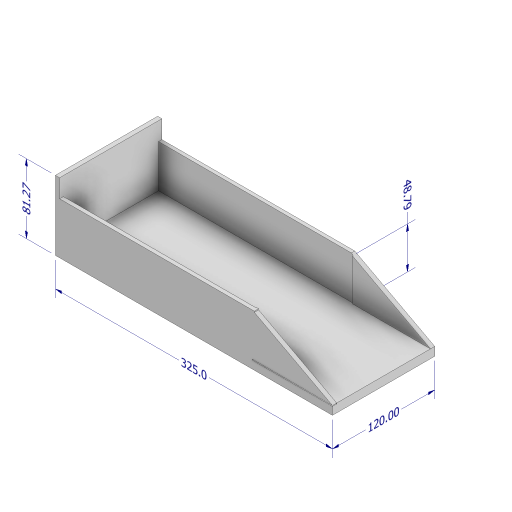
# Autodesk Inventor part: Storagecontainer
Saved by Autodesk Inventor 2024 (Build 280153000, 153)
## iProperties
Created: 2023-05-30
Part Number: Storagecontainer
Material: Generic
Document SubType Name: Modeling
Designer: Lenovo
Density: 1 g/cm^3
Appearance: Default
Author: Lenovo
Autodesk Inventor part; units mm, degrees
ref_plane "YZ Plane" through (0, 0, 0) normal (1, 0, 0) x (0, 1, 0)
ref_plane "XZ Plane" through (0, 0, 0) normal (0, 1, 0) x (-1, 0, 0)
ref_plane "XY Plane" through (0, 0, 0) normal (0, 0, 1) x (1, 0, 0)
sketch "Sketch1" plane through (0, 0, 0) normal (0, 1, 0) x (-1, 0, 0)
  line L0 (-160, 60) -> (160, 60)
  line L1 (160, 60) -> (160, -60)
  line L2 (160, -60) -> (-160, -60)
  line L3 (-160, -60) -> (-160, 60)
  line L4 (-160, 60) -> (160, -60) construction
  line L5 (160, 60) -> (-160, -60) construction
  line L6 (-27.6343, -87.1189) -> (-42.3128, -87.1189)
  line L7 (-42.3128, -87.1189) -> (-42.3128, -133.601)
  line L8 (-42.3128, -133.601) -> (-27.6343, -133.601)
  line L9 (-27.6343, -133.601) -> (-27.6343, -87.1189)
  line L10 (-27.6343, -87.1189) -> (-42.3128, -133.601) construction
  line L11 (-42.3128, -87.1189) -> (-27.6343, -133.601) construction
  point P0 (0, 0)
  point P1 (-34.9736, -110.3599)
  dimension "d0" = 320
  dimension "d1" = 120
  constraints: 24 end point, 4 midpoint, 4 parallel, 2 horizontal, 2 perpendicular
  measures "d0" distance of L1.end L2.end
  measures "d1" distance of L0.end L1.end
extrude "Extrusion1" add sketch "Sketch1" along normal blind 10 contours L0 L1 L2 L3
sketch "Sketch2" plane through (0, 10, 0) normal (0, 1, 0) x (1, 0, 0)
  line L0 (-160, -60) -> (160, -60) projected
  line L1 (-160, -60) -> (66.1592, -60)
  line L2 (66.1592, -60) -> (66.1592, -55.6043)
  line L3 (66.1592, -55.6043) -> (-160, -55.6043)
  line L4 (-160, -55.6043) -> (-160, -60)
  point P0 (0, 0)
  constraints: 8 end point, 2 parallel, 1 horizontal, 1 perpendicular
extrude "Extrusion2" add sketch "Sketch2" along normal blind 50
sketch "Sketch3" plane through (0, 10, 0) normal (0, 1, 0) x (1, 0, 0)
  line L0 (-160, 60) -> (-160, -60) projected
  line L1 (-160, 60) -> (68.4346, 60)
  line L2 (68.4346, 60) -> (68.4346, 56.0614)
  line L3 (68.4346, 56.0614) -> (-160, 56.0614)
  line L4 (-160, 56.0614) -> (-160, 60)
  point P0 (0, 0)
  constraints: 8 end point, 2 parallel, 1 horizontal, 1 perpendicular
extrude "Extrusion3" add sketch "Sketch3" along normal blind 50
sketch "Sketch4" plane through (-160, 0, -60) normal (-1, 0, 0) x (0, 0, 1)
  line L0 (120, -68.4573) -> (0, -68.4573)
  line L1 (0, -68.4573) -> (0, 81.272)
  line L2 (0, 81.272) -> (120, 81.272)
  line L3 (120, 81.272) -> (120, -68.4573)
  line L4 (120, -68.4573) -> (0, 81.272) construction
  line L5 (0, -68.4573) -> (120, 81.272) construction
  point P0 (60, 0)
  point P1 (60, 6.4073)
  constraints: 12 end point, 2 midpoint, 2 parallel, 1 horizontal, 1 perpendicular
extrude "Extrusion4" add sketch "Sketch4" along normal blind 5
sketch "Sketch5" plane through (-165, 0, -60) normal (-1, 0, 0) x (0, 0, 1)
  line L0 (120, -68.4573) -> (120, 81.272) projected
  line L1 (0, 0) -> (120, 0)
  line L2 (120, 0) -> (120, -68.4573)
  line L3 (120, -68.4573) -> (0, -68.4573)
  line L4 (0, -68.4573) -> (0, 0)
  point P0 (60, 0)
  constraints: 8 end point, 2 parallel, 1 horizontal, 1 perpendicular
extrude "Extrusion5" cut sketch "Sketch5" against normal blind 5
sketch "Sketch6" plane through (160, 0, -60) normal (0, 0, -1) x (-1, 0, 0)
  line L0 (91.5654, 10) -> (91.5654, 60) projected
  line L1 (0, 0) -> (0, 10) projected
  line L2 (91.5654, 60) -> (0, 60)
  line L3 (0, 60) -> (0, 10)
  line L4 (0, 10) -> (91.5654, 10)
  line L5 (91.5654, 10) -> (91.5654, 60)
  point P0 (160, 0)
  constraints: 8 end point, 2 parallel, 1 horizontal, 1 perpendicular
extrude "Extrusion6" add sketch "Sketch6" against normal blind 5
sketch "Sketch7" plane through (160, 0, 60) normal (0, 0, 1) x (1, 0, 0)
  line L0 (-93.8408, 10) -> (-93.8408, 60) projected
  line L1 (0, 0) -> (0, 60) projected
  line L2 (-93.8408, 60) -> (0, 60)
  line L3 (0, 60) -> (0, 9.1052)
  line L4 (0, 9.1052) -> (-93.8408, 9.1052)
  line L5 (-93.8408, 9.1052) -> (-93.8408, 60)
  point P0 (-160, 0)
  constraints: 8 end point, 2 parallel, 1 horizontal, 1 perpendicular, 1 point on line
extrude "Extrusion7" cut sketch "Sketch7" against normal blind 5
sketch "Sketch8" plane through (-160, 60, 60) normal (0, 0, 1) x (1, 0, 0)
  line L0 (320, -50) -> (228.4346, -50) projected
  line L1 (226.1592, 0) -> (320, 0)
  line L2 (320, 0) -> (320, -50)
  line L3 (320, -50) -> (226.1592, -50)
  line L4 (226.1592, -50) -> (226.1592, 0)
  point P0 (160, -60)
  constraints: 8 end point, 2 parallel, 1 horizontal, 1 perpendicular
extrude "Extrusion8" add sketch "Sketch8" against normal blind 5
sketch "Sketch9" plane through (160, 0, -60) normal (0, 0, -1) x (-1, 0, 0)
  line L0 (93.8408, 10) -> (93.8408, 60) projected
  line L1 (0, 10) -> (91.5654, 10) projected
  line L2 (93.8408, 60) -> (0, 10)
  line L3 (0, 10) -> (0, 60)
  line L4 (0, 60) -> (93.8408, 60)
  point P0 (160, 0)
  constraints: 6 end point, 2 perpendicular
extrude "Extrusion9" cut sketch "Sketch9" against normal blind 5
sketch "Sketch10" plane through (-160, 60, 55) normal (0, 0, -1) x (-1, 0, 0)
  point P0 (-160, -60)
sketch "Sketch11" plane through (-160, 60, 60) normal (0, 0, 1) x (1, 0, 0)
  line L0 (228.4346, -50) -> (228.4346, 0)
  line L1 (0, 0) -> (320, 0) projected
  line L2 (320, -50) -> (320, 0) projected
  line L3 (320, -50) -> (228.4346, -1.2124) projected
  line L4 (320, -50) -> (228.4346, -1.2124)
  line L5 (228.4346, -1.2124) -> (228.4346, -50)
  line L6 (320, -60) -> (-5, -60) projected
  point P0 (160, -60)
  constraints: 6 end point, 1 collinear, 1 perpendicular, 1 point on line, 1 vertical
extrude "Extrusion10" cut sketch "Sketch11" against normal blind 5
body "Solid1"
